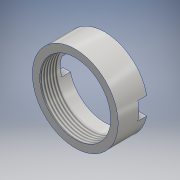
# Autodesk Inventor part: Bague Prise Banane
Saved by Autodesk Inventor 2016 SP1 (Build 200210100, 210)
## iProperties
Created: 2018-06-13
Part Number: Bague Prise Banane
Material: Aluminium 6061
Document SubType Name: Modeling
Designer: dimercur
Density: 2.7 g/cm^3
Appearance: Aluminium - Plat
Mass: 0.70244 g
Surface Area: 5.20326 cm^2
Volume: 0.260163 cm^3
Author: dimercur
Autodesk Inventor part; units mm, degrees
ref_plane "YZ Plane" through (0, 0, 0) normal (1, 0, 0) x (0, 1, 0)
ref_plane "XZ Plane" through (0, 0, 0) normal (0, 1, 0) x (-1, 0, 0)
ref_plane "XY Plane" through (0, 0, 0) normal (0, 0, 1) x (1, 0, 0)
sketch "Esquisse1" plane through (0, 0, 0) normal (0, 1, 0) x (-1, 0, 0)
  circle A0 centre (0, 0) radius 7.25
  circle A1 centre (0, 0) radius 6
  dimension "d0" = 12
  dimension "d1" = 14.5
  constraints: 2 centre point, 2 coincident
  measures "d0" diameter of A1
  measures "d1" diameter of A0
extrude "Extrusion1" add sketch "Esquisse1" along normal blind 5
sketch "Esquisse2" plane through (0, 5, 0) normal (0, 1, 0) x (1, 0, 0)
  line L0 (-8, -1.5) -> (-5, -1.5)
  line L1 (-5, -1.5) -> (-5, 1.5)
  line L2 (-5, 1.5) -> (-8, 1.5)
  line L3 (-8, 1.5) -> (-8, -1.5)
  line L4 (5, -1.5) -> (8, -1.5)
  line L5 (8, -1.5) -> (8, 1.5)
  line L6 (8, 1.5) -> (5, 1.5)
  line L7 (5, 1.5) -> (5, -1.5)
  point P0 (0, 0)
  dimension "d4" = 3
  dimension "d5" = 1.5
  dimension "d6" = 3
  dimension "d7" = 3
  dimension "d8" = 5
  dimension "d9" = 5
  constraints: 16 end point, 4 parallel, 2 horizontal, 2 perpendicular, 2 point on line
  measures "d4" distance of L2.end L0.start
  measures "d5" vertical distance of point (0, 0) L0.start
  measures "d6" distance of L0.start L0.end
  measures "d7" distance of L4.start L4.end
  measures "d8" distance from line of point (0, 0) L7
  measures "d9" distance from line of point (0, 0) L1
extrude "Extrusion2" cut sketch "Esquisse2" against normal blind 1.5
thread "Filetage1" size "M12x0.5" class "6H" standard "ANSI Metric M Profile" length 8 offset 2
equation "\"d5\" = 0.5 * d4"
equation "\"d9\" = d8"
